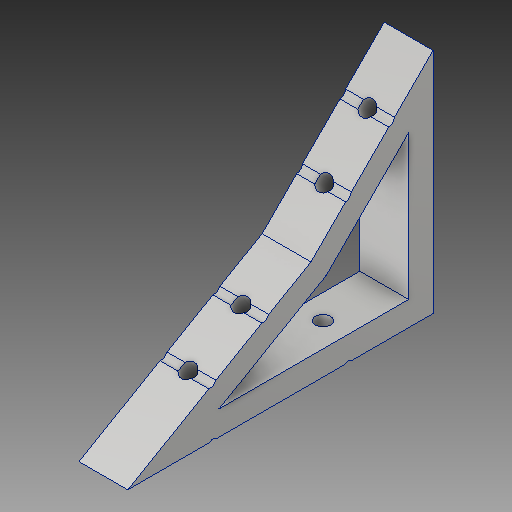
# Autodesk Inventor part: 칼팁중간받침대
Saved by Autodesk Inventor 2017 (Build 210142000, 142)
## iProperties
Part Number: 칼팁중간받침대
Material: 알루미늄 6061
Document SubType Name: Modeling
Designer: minom
Density: 2.7 g/cm^3
Appearance: 알루미늄 - 평지
Mass: 8.00982 g
Surface Area: 29.283 cm^2
Volume: 2.9666 cm^3
Author: minom
Autodesk Inventor part; units mm, degrees
ref_plane "YZ Plane" through (0, 0, 0) normal (1, 0, 0) x (0, 1, 0)
ref_plane "XZ Plane" through (0, 0, 0) normal (0, 1, 0) x (-1, 0, 0)
ref_plane "XY Plane" through (0, 0, 0) normal (0, 0, 1) x (1, 0, 0)
sketch "스케치1" plane through (0, 0, 0) normal (1, 0, 0) x (0, 1, 0)
  line L0 (0, 0) -> (0, 20)
  line L1 (0, 20) -> (0, 50)
  line L2 (0, 0) -> (37.3205, 0)
  line L3 (0, 20) -> (17.3205, 20)
  line L4 (0, 50) -> (17.3205, 20)
  line L5 (0, 50) -> (34.641, 50) construction
  line L6 (17.3205, 20) -> (37.3205, 0)
  line L7 (17.3205, 20) -> (45.6048, 20) construction
  dimension "d0" = 20
  dimension "d1" = 30
  dimension "d2" = 60
  dimension "d3" = 45
  constraints: 16 end point, 4 horizontal, 2 equal length, 1 point on line, 1 vertical
  measures "d0" distance of L0.start L0.end
  measures "d1" distance of L0.end L1.end
  measures "d2" angle of L4 L5
  measures "d3" angle of L6 L7
extrude "돌출1" add sketch "스케치1" along normal blind 8
sketch "스케치2" plane through (8, 0, 0) normal (1, 0, 0) x (0, 0, -1)
  line L0 (-20, 17.3205) -> (-50, 0) projected
  line L1 (-50, 0) -> (0, 0) projected
  line L2 (0, 0) -> (0, 37.3205) projected
  line L3 (0, 37.3205) -> (-20, 17.3205) projected
  line L4 (-35.0718, 4) -> (-17.5439, 14.1197)
  line L5 (-17.5439, 14.1197) -> (-4, 27.6637)
  line L6 (-4, 27.6637) -> (-4, 4)
  line L7 (-4, 4) -> (-35.0718, 4)
  dimension "d6" = 4
  constraints: 8 end point, 3 other
  measures "d6" distance between parallel lines of L0 L4
extrude "돌출2" cut sketch "스케치2" against normal blind 8 contours L4 L5 L6 L7
sketch "스케치5" plane through (0, 0, 0) normal (0, -1, 0) x (1, 0, 0)
  arc A0 (157.7, 33) -> (156.7, 34) centre (156.7, 33) ccw projected
  line L0 (157.7, 33) -> (157.7, 24) projected
  arc A1 (156.7, 23) -> (157.7, 24) centre (156.7, 24) ccw projected
  line L1 (156.7, 23) -> (136.7, 23) projected
  arc A2 (135.7, 24) -> (136.7, 23) centre (136.7, 24) ccw projected
  line L2 (135.7, 24) -> (135.7, 33) projected
  arc A3 (136.7, 34) -> (135.7, 33) centre (136.7, 33) ccw projected
  line L3 (136.7, 34) -> (156.7, 34) projected
  arc A4 (-61.9, 33) -> (-62.9, 34) centre (-62.9, 33) ccw projected
  line L4 (-61.9, 33) -> (-61.9, 24) projected
  arc A5 (-62.9, 23) -> (-61.9, 24) centre (-62.9, 24) ccw projected
  line L5 (-62.9, 23) -> (-82.9, 23) projected
  arc A6 (-83.9, 24) -> (-82.9, 23) centre (-82.9, 24) ccw projected
  line L6 (-83.9, 24) -> (-83.9, 33) projected
  arc A7 (-82.9, 34) -> (-83.9, 33) centre (-82.9, 33) ccw projected
  line L7 (-82.9, 34) -> (-62.9, 34) projected
  arc A8 (-61.9, -244) -> (-62.9, -243) centre (-62.9, -244) ccw projected
  line L8 (-61.9, -244) -> (-61.9, -253) projected
  arc A9 (-62.9, -254) -> (-61.9, -253) centre (-62.9, -253) ccw projected
  line L9 (-62.9, -254) -> (-82.9, -254) projected
  arc A10 (-83.9, -253) -> (-82.9, -254) centre (-82.9, -253) ccw projected
  line L10 (-83.9, -253) -> (-83.9, -244) projected
  arc A11 (-82.9, -243) -> (-83.9, -244) centre (-82.9, -244) ccw projected
  line L11 (-82.9, -243) -> (-62.9, -243) projected
  arc A12 (136.7, -243) -> (135.7, -244) centre (136.7, -244) ccw projected
  line L12 (136.7, -243) -> (156.7, -243) projected
  arc A13 (157.7, -244) -> (156.7, -243) centre (156.7, -244) ccw projected
  line L13 (157.7, -244) -> (157.7, -253) projected
  arc A14 (156.7, -254) -> (157.7, -253) centre (156.7, -253) ccw projected
  line L14 (156.7, -254) -> (136.7, -254) projected
  arc A15 (135.7, -253) -> (136.7, -254) centre (136.7, -253) ccw projected
  line L15 (135.7, -253) -> (135.7, -244) projected
  line L16 (-98.1, 40) -> (171.9, 40) projected
  line L17 (-98.1, 0) -> (-98.1, 40) projected
  line L18 (-58.1, 0) -> (-98.1, 0) projected
  line L19 (-58.1, -220) -> (-58.1, 0) projected
  line L20 (-98.1, -220) -> (-58.1, -220) projected
  line L21 (-98.1, -260) -> (-98.1, -220) projected
  line L22 (171.9, -260) -> (-98.1, -260) projected
  line L23 (171.9, -220) -> (171.9, -260) projected
  line L24 (131.9, -220) -> (171.9, -220) projected
  line L25 (131.9, 0) -> (131.9, -220) projected
  line L26 (171.9, 0) -> (131.9, 0) projected
  line L27 (171.9, 40) -> (171.9, 0) projected
  circle A16 centre (4, 14.0286) radius 1.25
  circle A17 centre (4, 36.0286) radius 1.25
  point P0 (0, 0)
  dimension "d17" = 2.5
  dimension "d18" = 2.5
  constraints: 2 centre point
  measures "d17" diameter of A16
  measures "d18" diameter of A17
extrude "돌출5" cut sketch "스케치5" against normal blind 4.1 contours A16 | A17
sketch "스케치8" plane through (0, 17.3205, 20) normal (0, 0.7071068, 0.7071068) x (1, 0, 0)
  circle A0 centre (4, 8.6869) radius 1.5
  circle A1 centre (4, 18.6869) radius 1.5
  circle A2 centre (4, 18.6869) radius 1.25
  circle A3 centre (4, 8.6869) radius 1.25
  point P0 (0, 1.8947)
  dimension "d35" = 2.5
  dimension "d36" = 2.5
  constraints: 4 centre point, 2 coincident, 4 other
  measures "d35" diameter of A2
  measures "d36" diameter of A3
extrude "돌출7" cut sketch "스케치8" against normal blind 4.1 contours A2 | A3
sketch "스케치9" plane through (0, 0, 50) normal (0, 0.8660254, 0.5) x (1, 0, 0)
  circle A0 centre (4, 26) radius 1.5
  circle A1 centre (4, 16) radius 1.5
  circle A2 centre (4, 26) radius 1.25
  circle A3 centre (4, 16) radius 1.25
  point P0 (0, 43.3013)
  dimension "d39" = 2.5
  dimension "d40" = 2.5
  constraints: 4 centre point, 2 coincident, 4 other
  measures "d39" diameter of A2
  measures "d40" diameter of A3
extrude "돌출8" cut sketch "스케치9" against normal blind 4.1 contours A2 | A3
sketch "스케치10" plane through (8, 0, 0) normal (1, 0, 0) x (0, 0, -1)
  line L0 (-35.037, 4.1) -> (-35.037, 4.1) projected
  line L1 (-35.0184, 4.0308) -> (-35.037, 4.1) projected
  line L2 (-35.0184, 4.0308) -> (-35.0184, 4.0308) projected
  line L3 (-35.037, 4.1) -> (-35.0184, 4.0308) projected
  line L4 (-37.2261, 7.375) -> (-35.0611, 8.625) projected
  line L5 (-24.4008, 10.1609) -> (-26.5659, 8.9109) projected
  line L6 (-28.5659, 12.375) -> (-26.4008, 13.625) projected
  line L7 (-10.1451, 21.5185) -> (-11.9129, 19.7508) projected
  line L8 (-14.7413, 22.5792) -> (-12.9735, 24.347) projected
  line L9 (-7.6702, 29.6503) -> (-5.9025, 31.418) projected
  line L10 (-4, 27.5222) -> (-4, 27.6637) projected
  line L11 (-4, 27.5222) -> (-4, 27.5222) projected
  line L12 (-4, 27.6637) -> (-4, 27.5222) projected
  line L13 (-4, 27.6637) -> (-4, 27.6637) projected
  line L14 (-15.2786, 4) -> (-12.7786, 4) projected
  line L15 (-12.7786, 0) -> (-15.2786, 0) projected
  line L16 (-35.037, 4.1) -> (-35.0184, 4.0308) projected
  line L17 (-35.0718, 4) -> (-35.0184, 4.0308) projected
  line L18 (-35.0102, 4) -> (-35.0718, 4) projected
  line L19 (-35.0102, 4) -> (-34.9916, 3.9308) projected
  line L20 (-34.9916, 3.9308) -> (-34.8718, 4) projected
  line L21 (-34.8718, 4) -> (-34.8718, 4) projected
  line L22 (-34.8718, 4) -> (-34.9916, 3.9308) projected
  line L23 (-34.9916, 3.9308) -> (-35.0102, 4) projected
  line L24 (-35.0718, 4) -> (-35.0102, 4) projected
  line L25 (-35.0184, 4.0308) -> (-35.0718, 4) projected
  line L26 (-35.0184, 4.0308) -> (-35.037, 4.1) projected
  line L27 (-35.037, 4.1) -> (-35.037, 4.1) projected
  line L28 (-34.7786, 0) -> (-37.2786, 0) projected
  arc A0 (-36.7164, 7.6693) -> (-35.5708, 8.3307) centre (-36.5186, 8.6495) ccw
  arc A1 (-28.0562, 12.6693) -> (-26.9105, 13.3307) centre (-27.8583, 13.6495) ccw
  arc A2 (-14.3251, 22.9954) -> (-13.3897, 23.9308) centre (-14.3878, 23.9934) ccw
  arc A3 (-7.2541, 30.0664) -> (-6.3187, 31.0019) centre (-7.3167, 31.0645) ccw
  arc A4 (-13.196, 0) -> (-14.5189, 0) centre (-13.8574, -0.75) ccw
  arc A5 (-35.3671, 0) -> (-36.69, 0) centre (-36.0286, -0.75) ccw
  point P0 (0, 0)
  dimension "d43" = 2
  dimension "d44" = 2
  dimension "d45" = 2
  dimension "d46" = 2
  dimension "d47" = 2
  dimension "d48" = 2
  dimension "d49" = 0.75
  dimension "d50" = 0.75
  dimension "d51" = 0.75
  dimension "d52" = 0.75
  dimension "d53" = 0.75
  dimension "d54" = 0.75
  constraints: 12 point on circle, 12 point on line, 6 centre point
  measures "d43" diameter of A0
  measures "d44" diameter of A1
  measures "d45" diameter of A2
  measures "d46" diameter of A3
  measures "d47" diameter of A4
  measures "d48" diameter of A5
  measures "d49" distance from line of L4 A0.centre
  measures "d50" distance from line of L6 A1.centre
  measures "d51" distance from line of L8 A2.centre
  measures "d52" distance from line of L9 A3.centre
  measures "d53" distance from line of L15 A4.centre
  measures "d54" distance from line of L28 A5.centre
extrude "돌출9" cut sketch "스케치10" against normal blind 8
